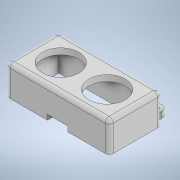
# Autodesk Inventor part: Part5
Saved by Autodesk Inventor 2022 (Build 260153000, 153)
## iProperties
Created: 2021-10-11
Part Number: Part5
Material: Generic
Document SubType Name: Modeling
Designer: Route
Density: 1 g/cm^3
Appearance: Default
Author: Route
Autodesk Inventor part; units mm, degrees
ref_plane "YZ Plane" through (0, 0, 0) normal (1, 0, 0) x (0, 1, 0)
ref_plane "XZ Plane" through (0, 0, 0) normal (0, 1, 0) x (-1, 0, 0)
ref_plane "XY Plane" through (0, 0, 0) normal (0, 0, 1) x (1, 0, 0)
sketch "Sketch1" plane through (0, 0, 0) normal (0, 1, 0) x (-1, 0, 0)
  line L0 (-77, 17) -> (-32, 17)
  line L1 (-32, 17) -> (-32, -3)
  line L2 (-32, -3) -> (-77, -3)
  line L3 (-77, -3) -> (-77, 17)
  line L4 (-78, 20) -> (-31, 20)
  line L5 (-29, 18) -> (-29, -4)
  line L6 (-41, -6) -> (-68, -6)
  line L7 (-80, -4) -> (-80, 18)
  arc A0 (-78, 20) -> (-80, 18) centre (-78, 18) ccw
  arc A1 (-29, 18) -> (-31, 20) centre (-31, 18) ccw
  arc A2 (-31, -6) -> (-29, -4) centre (-31, -4) ccw
  arc A3 (-80, -4) -> (-78, -6) centre (-78, -4) ccw
  line L8 (-77, -3) -> (-75.5, -3)
  line L9 (-75.5, -3) -> (-75.5, -1.5)
  circle A4 centre (-75.5, -1.5) radius 1
  line L10 (-32, 17) -> (-33.5, 17)
  line L11 (-33.5, 17) -> (-33.5, 15.5)
  circle A5 centre (-33.5, 15.5) radius 1
  line L12 (-49.42, 17) -> (-59.58, 17)
  line L13 (-59.58, 17) -> (-59.58, 14.46)
  line L14 (-59.58, 14.46) -> (-49.42, 14.46)
  line L15 (-49.42, 14.46) -> (-49.42, 17)
  line L16 (-78, -6) -> (-31, -6)
  line L17 (-77, -6) -> (-71, -6)
  line L18 (-71, -9) -> (-71, -9)
  line L19 (-74, -12) -> (-74, -12)
  line L20 (-77, -9) -> (-77, -6)
  line L21 (-32, -6) -> (-38, -6)
  line L22 (-38, -9) -> (-38, -9)
  line L23 (-35, -12) -> (-35, -12)
  line L24 (-32, -9) -> (-32, -6)
  arc A6 (-77, -9) -> (-74, -12) centre (-74, -9) ccw
  arc A7 (-74, -12) -> (-71, -9) centre (-74, -9) ccw
  arc A8 (-68, -6) -> (-71, -9) centre (-68, -9) ccw
  arc A9 (-38, -9) -> (-41, -6) centre (-41, -9) ccw
  arc A10 (-38, -9) -> (-35, -12) centre (-35, -9) ccw
  arc A11 (-35, -12) -> (-32, -9) centre (-35, -9) ccw
  circle A12 centre (-74, -9) radius 1.5
  circle A13 centre (-35, -9) radius 1.5
  line L25 (-77, -6) -> (-68, -6)
  line L26 (-41, -6) -> (-32, -6)
  point P0 (0, 0)
  point P1 (-38, -12)
  dimension "d44" = 45
  dimension "d45" = 20
  dimension "d46" = 2
  dimension "d47" = 1.5
  dimension "d48" = 1.5
  dimension "d49" = 2
  dimension "d50" = 1.5
  dimension "d51" = 1.5
  dimension "d52" = 2
  dimension "d53" = 10.16
  dimension "d54" = 2.54
  dimension "d55" = 3
  dimension "d56" = 3
  dimension "d57" = 3
  constraints: 54 end point, 20 point on circle, 20 tangent, 14 centre point, 13 point on line, 9 perpendicular, 8 equal radius, 8 parallel, 4 coincident, 4 horizontal, 2 collinear
  measures "d44" distance of L2.start L2.end
  measures "d45" distance of L0.end L2.start
  measures "d46" radius of A0
  measures "d47" distance of L2.end L9.start
  measures "d48" distance of L9.start L9.end
  measures "d49" diameter of A4
  measures "d50" distance of L0.end L11.start
  measures "d51" distance of L11.start L11.end
  measures "d52" diameter of A5
  measures "d53" distance of L12.start L13.start
  measures "d54" distance of L13.start L13.end
  measures "d55" radius of A6
  measures "d56" diameter of A12
  measures "d57" diameter of A13
extrude "Extrusion1" add sketch "Sketch1" along normal blind 3 contours L4 A1 L5 A2 L16 L6 A3 L7 A0 | L16 A8 A7 A6 L20 | L24 A11 A10 A9 L16
sketch "Sketch2" plane through (0, 3, 0) normal (0, 1, 0) x (1, 0, 0)
  line L0 (32, 3) -> (77, 3) projected
  line L1 (77, -17) -> (32, -17) projected
  line L2 (32, 3) -> (77, 3)
  line L3 (77, 3) -> (77, -17)
  line L4 (77, -17) -> (32, -17)
  line L5 (32, -17) -> (32, 3)
  line L6 (31, 6) -> (78, 6)
  line L7 (80, 4) -> (80, -18)
  line L8 (78, -20) -> (31, -20)
  line L9 (29, -18) -> (29, 4)
  arc A0 (31, 6) -> (29, 4) centre (31, 4) ccw
  arc A1 (80, 4) -> (78, 6) centre (78, 4) ccw
  arc A2 (78, -20) -> (80, -18) centre (78, -18) ccw
  arc A3 (29, -18) -> (31, -20) centre (31, -18) ccw
  point P0 (0, 0)
  dimension "d60" = 2
  constraints: 16 end point, 8 point on circle, 8 tangent, 4 centre point, 4 parallel, 3 equal radius, 2 horizontal, 2 perpendicular
  measures "d60" radius of A0
extrude "Extrusion2" add sketch "Sketch2" along normal blind 9
sketch "Sketch3" plane through (0, 12, 0) normal (0, 1, 0) x (1, 0, 0)
  line L0 (31, 6) -> (78, 6)
  line L1 (80, 4) -> (80, -18)
  line L2 (78, -20) -> (31, -20)
  line L3 (29, -18) -> (29, 4)
  arc A0 (31, 6) -> (29, 4) centre (31, 4) ccw
  arc A1 (80, 4) -> (78, 6) centre (78, 4) ccw
  arc A2 (78, -20) -> (80, -18) centre (78, -18) ccw
  arc A3 (29, -18) -> (31, -20) centre (31, -18) ccw
  point P0 (0, 0)
  dimension "d63" = 2
  constraints: 8 end point, 8 point on circle, 8 tangent, 4 centre point, 3 equal radius, 2 parallel, 1 horizontal, 1 perpendicular
  measures "d63" radius of A0
extrude "Extrusion3" add sketch "Sketch3" along normal blind 3
fillet "Fillet1" radius 2 8 edges at (29.5858, 15, -5.4142) (29, 15, 7) (29.5858, 15, 19.4142) (54.5, 15, 20) (79.4142, 15, 19.4142) (80, 15, 7) (79.4142, 15, -5.4142) (54.5, 15, -6)
sketch "Sketch4" plane through (0, 0, 0) normal (0, -1, 0) x (1, 0, 0)
  line L0 (31, 20) -> (78, 20) projected
  line L1 (54.5, 20) -> (49.42, 20)
  line L2 (49.42, 20) -> (59.58, 20)
  line L3 (59.58, 20) -> (59.58, 17)
  line L4 (77, 17) -> (32, 17) projected
  line L5 (49.42, 20) -> (49.42, 17)
  line L6 (49.42, 17) -> (59.58, 17)
  point P0 (0, 0)
  dimension "d67" = 5.08
  dimension "d68" = 10.16
  constraints: 10 end point, 3 point on line, 2 perpendicular, 1 midpoint, 1 vertical
  measures "d67" distance of L1.start L1.end
  measures "d68" distance of L1.end L2.end
extrude "Extrusion4" cut sketch "Sketch4" against normal blind 2.54
sketch "Sketch5" plane through (0, 15, 0) normal (0, 1, 0) x (1, 0, 0)
  line L0 (78, -18) -> (31, -18) projected
  line L1 (31, 4) -> (78, 4) projected
  circle A0 centre (43, -7) radius 9
  circle A1 centre (66, -7) radius 9
  point P0 (0, 0)
  constraints: 2 centre point
extrude "Extrusion5" cut sketch "Sketch5" against normal blind 3
body "Solid1"
